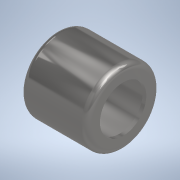
# Autodesk Inventor part: HK0609FMSH
Saved by Autodesk Inventor 2021.3 (Build 253353000, 353)
## iProperties
Part Number: HK0609FMSH
Material: 一般
Catalog Web Link: www.cadenas.de
Description: Needle Roller Shell Bearings open-ended SH-
Vendor: NTN
Document SubType Name: Modeling
Designer: partserver
Manufacturer: NTN
Mass: 0.159503 g
Surface Area: 6.5885 cm^2
Volume: 0.159503 cm^3
Density: 1 g/cm^3
Appearance: ステンレス - ブラシ仕上げ
Category: PARTsolutions
Company: NTN
PSOL_IDENT_0: {$CADENAS_DATA\23d-libs\ntn\needle_roler_bearings\needle_roller_shell_bearings_open_ended.prj},196 {
PSOL_IDENT_1: VTYP=3D},{NB=HK0609FMSH},{LINA=HK0609FMSH},{NN=Needle Roller Shell Bearings open-ended SH},{DATE=23.
PSOL_IDENT_2: 10.2020 01:12:36},{GEOMDATE=20.04.2020 08:31:59},{VERSION=},{LINEID=40},{WBVAR=},{WBNUMERIC=}  {NB=H
PSOL_IDENT_3: K0609FMSH},{LINA=HK0609FMSH},{KT=DUMMY},{FW=6},{D=10.0},{C=9},{ORDER=HK0609FM},{CR=2920},{COR=2590},
PSOL_IDENT_4: {CRF=298},{CORF=264},{LSG=25000},{LSO=37000},{MASS=0.0022},{IT=-},{RT=1.6},{VER=1},{T=0.500},{DW=1.5
PSOL_IDENT_5: 00},{LW=5.000},{NR=9.000},{CID=6.750},{CD=8.250},{CW=7.600},{SD=6.300}
NB: HK0609FMSH
NN: Needle Roller Shell Bearings open-ended SH
NBSYN: $ORDER.SH
LINA: HK0609FMSH
CATALOG: NTN Corporation
FW: 6
D: 10
C: 9
ORDER: HK0609FM
CR: 2920
COR: 2590
CRF: 298
CORF: 264
LSG: 25000
LSO: 37000
MASS: 0.0022
IT: -
SUPPLIER: NTN
ARTICLENO: HK0609FMSH
BOMINFO: HK0609FMSH
CREATOR: CADENAS GmbH
Title: HK0609FMSH
Author: Cadenas PARTsolutions
Autodesk Inventor part; units mm, degrees
sketch "Sketch_1" plane through (0, 0, 0) normal (0, 0, 1) x (1, 0, 0)
  line L0 (9, 0) -> (0, 0)
  line L1 (0, 3.15) -> (0.5, 3.15)
  line L2 (0.5, 3.15) -> (0.5, 4.2)
  arc A0 (0.8, 4.5) -> (0.5, 4.2) centre (0.8, 4.2) ccw
  line L3 (0.8, 4.5) -> (8.2, 4.5)
  arc A1 (8.5, 4.2) -> (8.2, 4.5) centre (8.2, 4.2) ccw
  line L4 (8.5, 4.2) -> (8.5, 3.15)
  line L5 (8.5, 3.15) -> (9, 3.15)
  line L6 (9, 3.15) -> (9, 4.2)
  arc A2 (9, 4.2) -> (8.2, 5) centre (8.2, 4.2) ccw
  line L7 (8.2, 5) -> (0.8, 5)
  arc A3 (0.8, 5) -> (0, 4.2) centre (0.8, 4.2) ccw
  line L8 (0, 4.2) -> (0, 3.15)
  constraints: 18 end point, 8 point on circle, 4 centre point
revolve "Revolution1" add sketch "Sketch_1" angle 360 about axis through (9, 0, 0) along (1, 0, 0)
ref_plane "IP_1_XY" through (0, 0, 0) normal (1, 0, 0) x (0, 0, -1)
ref_plane "IP_1_YZ" through (0, 0, 0) normal (0, 0, -1) x (0, 1, 0)
ref_plane "IP_1_ZX" through (0, 0, 0) normal (0, 1, 0) x (1, 0, 0)
ref_plane "IP_5_XY" through (4.5, 0, 0) normal (1, 0, 0) x (0, 0, -1)
ref_plane "IP_5_YZ" through (4.5, 0, 0) normal (0, 0, -1) x (0, 1, 0)
ref_plane "IP_5_ZX" through (4.5, 0, 0) normal (0, 1, 0) x (1, 0, 0)
ref_plane "IP_6_XY" through (6.35, 0, 0) normal (1, 0, 0) x (0, 0, -1)
ref_plane "IP_6_YZ" through (6.35, 0, 0) normal (0, 0, -1) x (0, 1, 0)
ref_plane "IP_6_ZX" through (6.35, 0, 0) normal (0, 1, 0) x (1, 0, 0)
body "Solid1"
